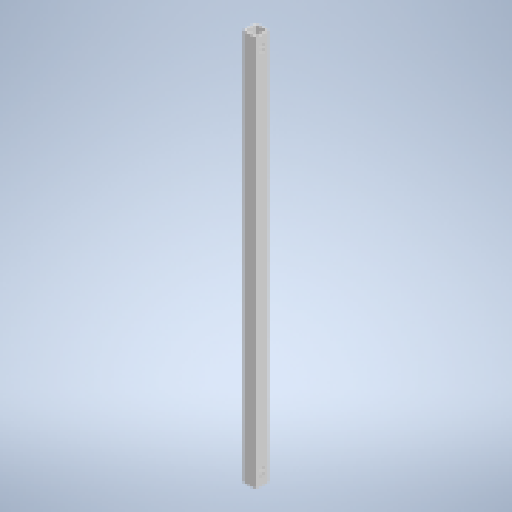
# Autodesk Inventor part: 15x15x455
Saved by Autodesk Inventor 2025.2 (Build 292293000, 293)
## iProperties
Created: 2025-03-27
Part Number: 15x15x455
Material: Generic
Document SubType Name: Modeling
Designer: Zhopa
Density: 1 g/cm^3
Appearance: Default
Author: Zhopa
Autodesk Inventor part; units mm, degrees
ref_plane "YZ Plane" through (0, 0, 0) normal (1, 0, 0) x (0, 1, 0)
ref_plane "XZ Plane" through (0, 0, 0) normal (0, 1, 0) x (-1, 0, 0)
ref_plane "XY Plane" through (0, 0, 0) normal (0, 0, 1) x (1, 0, 0)
sketch "Sketch1" plane through (0, 0, 0) normal (0, 1, 0) x (-1, 0, 0)
  line L0 (7.5, 7.5) -> (-7.5, 7.5)
  line L1 (-7.5, 7.5) -> (-7.5, -7.5)
  line L2 (-7.5, -7.5) -> (7.5, -7.5)
  line L3 (7.5, -7.5) -> (7.5, 7.5)
  line L4 (7.5, 7.5) -> (-7.5, -7.5) construction
  line L5 (-7.5, 7.5) -> (7.5, -7.5) construction
  line L6 (6, 6) -> (-6, 6)
  line L7 (-6, 6) -> (-6, -6)
  line L8 (-6, -6) -> (6, -6)
  line L9 (6, -6) -> (6, 6)
  line L10 (6, 6) -> (-6, -6) construction
  line L11 (-6, 6) -> (6, -6) construction
  point P0 (0, 0)
  dimension "d0" = 15
  dimension "d1" = 15
  dimension "d2" = 12
  dimension "d3" = 12
  constraints: 24 end point, 4 midpoint, 4 parallel, 2 horizontal, 2 perpendicular
  measures "d0" distance of L2.end L1.end
  measures "d1" distance of L1.end L0.end
  measures "d2" distance of L8.end L7.end
  measures "d3" distance of L7.end L6.end
extrude "Extrusion1" add sketch "Sketch1" along normal blind 455
sketch "Sketch2" plane through (7.5, 0, 7.5) normal (1, 0, 0) x (0, 0, -1)
  line L0 (0, 0) -> (15, 0) projected
  line L1 (0, 455) -> (15, 455) projected
  line L2 (0, 0) -> (0, 455) projected
  point P0 (7.5, 0)
  point P1 (7.5, 10)
  point P2 (7.5, 445)
  point P3 (7.5, 227.5)
  point P4 (7.5, 0)
  point P5 (7.5, 455)
  point P6 (7.5, 438)
  point P7 (7.5, 17)
  point P8 (7.5, 443.731)
  dimension "d6" = 10
  dimension "d8" = 227.5
  dimension "d9" = 455
  dimension "d10" = 210.5
  dimension "d11" = 210.5
  dimension "d19" = 433.731
  dimension "d20" = 7.5
  constraints: 2 midpoint
  measures "d6" distance from line of L0 point (7.5, 10)
  measures "d8" distance from line of point (7.5, 227.5) L1
  measures "d9" distance of point (7.5, 0) point (7.5, 455)
  measures "d10" distance of point (7.5, 227.5) point (7.5, 438)
  measures "d11" distance of point (7.5, 17) point (7.5, 227.5)
  measures "d19" distance of point (7.5, 10) point (7.5, 443.731)
  measures "d20" distance from line of L2 point (7.5, 443.731)
hole "Hole1" at (7.5, 10, 0) at (7.5, 438, 0) at (7.5, 17, 0) at (7.5, 443.731, 0) direction (-1, 0, 0) diameter 3.2 depth 80.45
equation "\"d8\" = 0.5 * d9"
body "Solid1"
